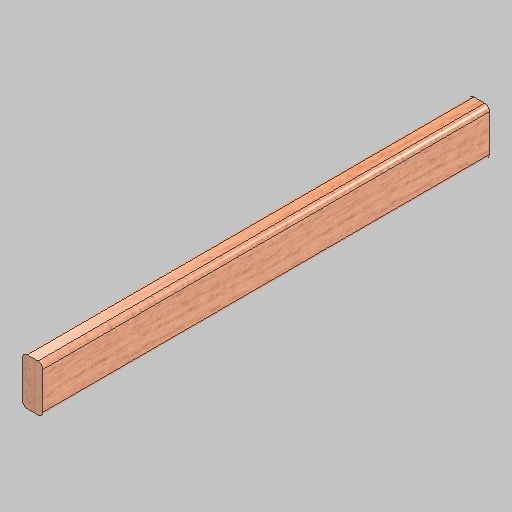
# Autodesk Inventor part: Ripas - Base - 458 mm
Saved by Autodesk Inventor 2025.2 (Build 292293000, 293)
## iProperties
Created: 2024-04-26
Part Number: Ripas - Base - 458 mm
Material: Genérico
Document SubType Name: Modeling
Designer: phmca
Density: 1 g/cm^3
Appearance: Padrão
Author: phmca
Autodesk Inventor part; units mm, degrees
ref_plane "YZ Plane" through (0, 0, 0) normal (1, 0, 0) x (0, 1, 0)
ref_plane "XZ Plane" through (0, 0, 0) normal (0, 1, 0) x (-1, 0, 0)
ref_plane "XY Plane" through (0, 0, 0) normal (0, 0, 1) x (1, 0, 0)
sketch "Esboço1" plane through (0, 0, 0) normal (0, 0, 1) x (1, 0, 0)
  line L0 (-5.5, 24) -> (5.5, 24)
  line L1 (10.5, 19) -> (10.5, -19)
  line L2 (5.5, -24) -> (-5.5, -24)
  line L3 (-10.5, -19) -> (-10.5, 19)
  line L4 (-10.5, 24) -> (10.5, -24) construction
  line L5 (10.5, 24) -> (-10.5, -24) construction
  arc A0 (-5.5, 24) -> (-10.5, 19) centre (-5.5, 19) ccw
  arc A1 (10.5, 19) -> (5.5, 24) centre (5.5, 19) ccw
  arc A2 (5.5, -24) -> (10.5, -19) centre (5.5, -19) ccw
  arc A3 (-10.5, -19) -> (-5.5, -24) centre (-5.5, -19) ccw
  point P0 (0, 0)
  dimension "d0" = 21
  dimension "d1" = 48
  dimension "d2" = 5
  constraints: 12 end point, 8 point on circle, 8 point on line, 8 tangent, 4 centre point, 3 equal radius, 2 midpoint, 2 parallel, 1 horizontal, 1 perpendicular
  measures "d0" distance of L4.end L5.end
  measures "d1" distance of L5.start L4.end
  measures "d2" radius of A0
extrude "Extrusão1" add sketch "Esboço1" along normal mid plane 458
